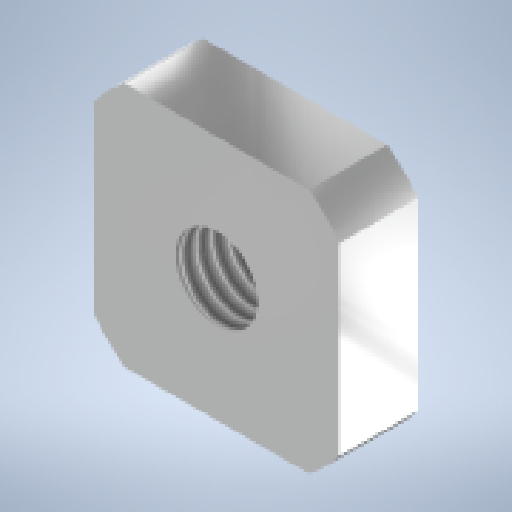
# Autodesk Inventor part: Levelling Foot Locknut
Saved by Autodesk Inventor 2024 (Build 280153000, 153)
## iProperties
Created: 2024-10-28
Part Number: Levelling Foot Locknut
Material: Aluminum 6061
Document SubType Name: Modeling
Designer: Ishaan
Density: 2.7 g/cm^3
Appearance: Aluminum - Flat
Author: Ishaan
Autodesk Inventor part; units mm, degrees
ref_plane "YZ Plane" through (0, 0, 0) normal (1, 0, 0) x (0, 1, 0)
ref_plane "XZ Plane" through (0, 0, 0) normal (0, 1, 0) x (-1, 0, 0)
ref_plane "XY Plane" through (0, 0, 0) normal (0, 0, 1) x (1, 0, 0)
sketch "Sketch1" plane through (0, 0, 0) normal (0, 0, 1) x (1, 0, 0)
  circle A0 centre (0, 0) radius 12.5
  line L0 (10, -12.5) -> (-10, -12.5)
  line L1 (-10, -12.5) -> (-10, 12.5)
  line L2 (-10, 12.5) -> (10, 12.5)
  line L3 (10, 12.5) -> (10, -12.5)
  line L4 (10, -12.5) -> (-10, 12.5) construction
  line L5 (-10, -12.5) -> (10, 12.5) construction
  line L6 (12.5, -10) -> (-12.5, -10)
  line L7 (-12.5, -10) -> (-12.5, 10)
  line L8 (-12.5, 10) -> (12.5, 10)
  line L9 (12.5, 10) -> (12.5, -10)
  line L10 (12.5, -10) -> (-12.5, 10) construction
  line L11 (-12.5, -10) -> (12.5, 10) construction
  point P0 (7.5, 10)
  point P1 (-7.5, 10)
  point P2 (-10, 7.5)
  point P3 (-10, -7.5)
  point P4 (-7.5, -10)
  point P5 (7.5, -10)
  point P6 (10, -7.5)
  point P7 (10, 7.5)
  dimension "d0" = 25
  dimension "d1" = 20
  constraints: 24 end point, 4 midpoint, 4 parallel, 3 perpendicular, 2 horizontal, 2 tangent, 1 centre point, 1 coincident
  measures "d0" diameter of A0
  measures "d1" distance of L1.end L2.end
extrude "Extrusion1" add sketch "Sketch1" along normal blind 6.35 contours L3 A0 L6 L1 L8
sketch "Sketch2" plane through (0, 0, 6.35) normal (0, 0, 1) x (1, 0, 0)
  arc A0 (-10, -7.5) -> (-7.5, -10) centre (0, 0) ccw projected
  constraints: 1 coincident
hole "Hole1" at (0, 0, 6.35) direction (0, 0, -1) diameter 6.647 end through all thread size "M8x1.25" class "6H" standard "ANSI Metric M Profile"
body "Solid1"
